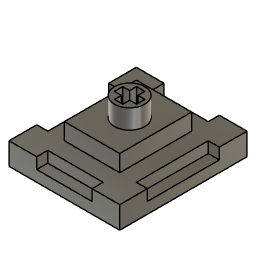
あa (Autodesk Fusion 360 design; units mm, degrees)
Autodesk Fusion 360 part; units mm, degrees
sketch "スケッチ1" plane through (0, 0, 0) normal (0, 0, 1) x (1, 0, 0)
  line L0 (0, 0) -> (20, 0)
  line L1 (20, 0) -> (20, 23)
  line L2 (20, 23) -> (0, 23)
  line L3 (0, 23) -> (0, 0)
  dimension "d1" = 20
  dimension "d2" = 23
  constraint horizontal L0
  constraint vertical L1
  constraint horizontal L2
  constraint vertical L3
  constraint coincident L0.start L3.end
  measures "d1" distance of L0.start L0.end
  measures "d2" distance of L0.start L2.end
extrude "押し出し1" add sketch "スケッチ1" along normal blind 2
sketch "スケッチ2" plane through (0, 0, 2) normal (0, 0, 1) x (-1, 0, 0)
  line L0 (0, -23) -> (0, 0)
  line L1 (0, 0) -> (-20, 0)
  line L2 (-20, 0) -> (-20, -23)
  line L3 (-20, -23) -> (0, -23)
  line L4 (0, -23) -> (-5, -23)
  line L5 (-5, -23) -> (-5, -18)
  line L6 (-5, -18) -> (0, -18)
  line L7 (0, -18) -> (0, -23)
  line L8 (-20, -23) -> (-15, -23)
  line L9 (-15, -23) -> (-15, -18)
  line L10 (-15, -18) -> (-20, -18)
  line L11 (-20, -18) -> (-20, -23)
  line L12 (0, 0) -> (-5, 0)
  line L13 (-5, 0) -> (-5, -5)
  line L14 (-5, -5) -> (0, -5)
  line L15 (0, -5) -> (0, 0)
  line L16 (-20, 0) -> (-15, 0)
  line L17 (-15, 0) -> (-15, -5)
  line L18 (-15, -5) -> (-20, -5)
  line L19 (-20, -5) -> (-20, 0)
  line L20 (-2, -21) -> (-18, -21)
  line L21 (-18, -21) -> (-18, -2)
  line L22 (-18, -2) -> (-2, -2)
  line L23 (-2, -2) -> (-2, -21)
  dimension "d5" = 5
  dimension "d6" = 5
  dimension "d7" = 5
  dimension "d8" = 5
  dimension "d9" = 5
  dimension "d10" = 5
  dimension "d11" = 5
  dimension "d12" = 5
  constraint horizontal L4
  constraint vertical L5
  constraint horizontal L6
  constraint vertical L7
  constraint coincident L0.start L3.end
  constraint horizontal L8
  constraint vertical L9
  constraint horizontal L10
  constraint vertical L11
  constraint coincident L2.end L3.start
  constraint horizontal L12
  constraint vertical L13
  constraint horizontal L14
  constraint vertical L15
  constraint coincident L0.end L1.start
  constraint horizontal L16
  constraint vertical L17
  constraint horizontal L18
  constraint vertical L19
  constraint coincident L1.end L2.start
  constraint horizontal L20
  constraint vertical L21
  constraint horizontal L22
  constraint vertical L23
  measures "d5" distance of L0.start L4.end
  measures "d6" distance of L0.start L6.end
  measures "d7" distance of L2.end L8.end
  measures "d8" distance of L2.end L10.end
  measures "d9" distance of L0.end L12.end
  measures "d10" distance of L0.end L14.end
  measures "d11" distance of L1.end L16.end
  measures "d12" distance of L1.end L18.end
extrude "押し出し2" add sketch "スケッチ2" along normal blind 2 contours L0 L3 L4 L5 L6 L7 L20 L23 | L0 L1 L12 L13 L14 L15 L22 L23 | L5 L6 L20 L23 | L5 L6 L9 L10 L13 L14 L17 L18 L20 L21 L22 L23 | L2 L3 L8 L9 L10 L11 L20 L21 | L13 L14 L22 L23 | L9 L10 L20 L21 | L1 L2 L16 L17 L18 L19 L21 L22 | L17 L18 L21 L22
sketch "スケッチ3" plane through (0, 0, 4) normal (0, 0, 1) x (-1, 0, 0)
  line L0 (-18, -18) -> (-20, -18)
  line L1 (-20, -18) -> (-20, -23)
  line L2 (-20, -23) -> (-15, -23)
  line L3 (-15, -23) -> (-15, -21)
  line L4 (-15, -21) -> (-5, -21)
  line L5 (-5, -21) -> (-5, -23)
  line L6 (-5, -23) -> (0, -23)
  line L7 (0, -23) -> (0, -18)
  line L8 (0, -18) -> (-2, -18)
  line L9 (-2, -18) -> (-2, -5)
  line L10 (-2, -5) -> (0, -5)
  line L11 (0, -5) -> (0, 0)
  line L12 (0, 0) -> (-5, 0)
  line L13 (-5, 0) -> (-5, -2)
  line L14 (-5, -2) -> (-15, -2)
  line L15 (-15, -2) -> (-15, 0)
  line L16 (-15, 0) -> (-20, 0)
  line L17 (-20, 0) -> (-20, -5)
  line L18 (-20, -5) -> (-18, -5)
  line L19 (-18, -5) -> (-18, -18)
  line L20 (-5, -18) -> (-15, -18)
  line L21 (-15, -18) -> (-15, -5)
  line L22 (-15, -5) -> (-5, -5)
  line L23 (-5, -5) -> (-5, -18)
  constraint horizontal L20
  constraint vertical L21
  constraint horizontal L22
  constraint vertical L23
extrude "押し出し3" add sketch "スケッチ3" along normal blind 3 contours L20 L21 L22 L23
sketch "スケッチ4" plane through (0, 0, 7) normal (0, 0, 1) x (-1, 0, 0)
  line L0 (-5, -5) -> (-15, -5)
  line L1 (-15, -5) -> (-15, -18)
  line L2 (-15, -18) -> (-5, -18)
  line L3 (-5, -18) -> (-5, -5)
  line L4 (-9.55, -13.5) -> (-11.05, -13.5)
  line L5 (-11.05, -13.5) -> (-11.05, -9.5)
  line L6 (-11.05, -9.5) -> (-9.55, -9.5)
  line L7 (-9.55, -9.5) -> (-9.55, -13.5)
  line L8 (-8.3, -12.25) -> (-12.3, -12.25)
  line L9 (-12.3, -12.25) -> (-12.3, -10.75)
  line L10 (-12.3, -10.75) -> (-8.3, -10.75)
  line L11 (-8.3, -10.75) -> (-8.3, -12.25)
  circle A0 centre (-10.3, -11.5) radius 2.75
  dimension "d17" = 13
  dimension "d18" = 1.5
  dimension "d19" = 4
  dimension "d20" = 4
  dimension "d21" = 1.5
  dimension "d22" = 5.5
  constraint horizontal L4
  constraint vertical L5
  constraint horizontal L6
  constraint vertical L7
  constraint horizontal L8
  constraint vertical L9
  constraint horizontal L10
  constraint vertical L11
  measures "d17" distance of L0 L2
  measures "d18" distance of L4.start L4.end
  measures "d19" distance of L4.start L6.end
  measures "d20" distance of L8.start L8.end
  measures "d21" distance of L8.start L10.end
  measures "d22" diameter of A0
extrude "押し出し4" add sketch "スケッチ4" along normal blind 3.5 contours A0
sketch "スケッチ5" plane through (0, 0, 0) normal (0, 0, -1) x (1, 0, 0)
  line L0 (0, 0) -> (0, -23)
  line L1 (0, -23) -> (20, -23)
  line L2 (20, -23) -> (20, 0)
  line L3 (20, 0) -> (0, 0)
  line L4 (20, -5) -> (0, -5) construction
  line L5 (0, -5) -> (0, -20) construction
  line L6 (0, -20) -> (20, -20) construction
  line L7 (20, -20) -> (20, -5) construction
  spline S0 degree 2 poles (12.4, -9.2465) (10.8153, -9.4071) (10.308, -9.915) knots 0 0 0 1 1 1
  spline S1 degree 2 poles (10.308, -9.915) (9.9278, -10.2946) (9.9278, -11.0222) knots 0 0 0 1 1 1
  spline S2 degree 2 poles (9.9278, -11.0222) (9.9278, -11.7963) (10.308, -12.1759) knots 0 0 0 1 1 1
  spline S3 degree 2 poles (10.308, -12.1759) (10.7658, -12.6343) (11.4922, -12.7053) knots 0 0 0 1 1 1
  spline S4 degree 2 poles (11.4922, -12.7053) (12.0723, -10.8115) (12.8076, -10.057) knots 0 0 0 1 1 1
  line L8 (12.8076, -10.057) -> (12.5826, -9.5581)
  line L9 (12.5826, -9.5581) -> (13.4558, -8.96)
  line L10 (13.4558, -8.96) -> (13.6391, -9.3718)
  spline S5 degree 2 poles (13.6391, -9.3718) (14.5284, -8.5482) (15.244, -8.5482) knots 0 0 0 1 1 1
  spline S6 degree 2 poles (15.244, -8.5482) (15.7436, -8.5482) (16.1507, -8.9546) knots 0 0 0 1 1 1
  spline S7 degree 2 poles (16.1507, -8.9546) (16.5947, -9.3993) (16.5947, -10.1609) knots 0 0 0 1 1 1
  spline S8 degree 2 poles (16.5947, -10.1609) (16.5947, -11.4555) (15.7012, -12.3496) knots 0 0 0 1 1 1
  spline S9 degree 2 poles (15.7012, -12.3496) (15.179, -12.8712) (14.6454, -13.156) knots 0 0 0 1 1 1
  line L11 (14.6454, -13.156) -> (14.572, -14.4285)
  line L12 (14.572, -14.4285) -> (16.1256, -14.3533)
  line L13 (16.1256, -14.3533) -> (16.2951, -15.3649)
  line L14 (16.2951, -15.3649) -> (14.532, -15.4019)
  spline S10 degree 2 poles (14.532, -15.4019) (14.4974, -16.1982) (14.4156, -17.0535) knots 0 0 0 1 1 1
  line L15 (14.4156, -17.0535) -> (13.5865, -17.0535)
  spline S11 degree 2 poles (13.5865, -17.0535) (13.1073, -16.9341) (13.4141, -16.6136) knots 0 0 0 1 1 1
  spline S12 degree 2 poles (13.4141, -16.6136) (13.4839, -15.9851) (13.5191, -15.4813) knots 0 0 0 1 1 1
  spline S13 degree 2 poles (13.5191, -15.4813) (11.8628, -15.553) (10.4662, -15.8186) knots 0 0 0 1 1 1
  line L16 (10.4662, -15.8186) -> (10.2978, -14.7794)
  spline S14 degree 2 poles (10.2978, -14.7794) (11.9661, -14.5789) (13.5651, -14.5072) knots 0 0 0 1 1 1
  line L17 (13.5651, -14.5072) -> (13.6313, -13.5338)
  spline S15 degree 2 poles (13.6313, -13.5338) (13.2535, -13.6806) (12.3874, -13.7158) knots 0 0 0 1 1 1
  line L18 (12.3874, -13.7158) -> (12.2711, -14.358)
  line L19 (12.2711, -14.358) -> (11.4474, -14.2064)
  spline S16 degree 2 poles (11.4474, -14.2064) (11.0099, -14.0877) (11.2797, -13.7725) knots 0 0 0 1 1 1
  line L20 (11.2797, -13.7725) -> (11.3095, -13.6334)
  spline S17 degree 2 poles (11.3095, -13.6334) (10.1988, -13.5272) (9.5458, -12.8736) knots 0 0 0 1 1 1
  spline S18 degree 2 poles (9.5458, -12.8736) (8.7997, -12.1282) (8.7997, -10.9846) knots 0 0 0 1 1 1
  spline S19 degree 2 poles (8.7997, -10.9846) (8.7997, -9.8875) (9.4706, -9.2173) knots 0 0 0 1 1 1
  spline S20 degree 2 poles (9.4706, -9.2173) (10.1713, -8.5165) (11.858, -8.2486) knots 0 0 0 1 1 1
  line L21 (11.858, -8.2486) -> (12.4, -9.2465)
  spline S21 degree 2 poles (14.523, -12.2183) (14.6525, -12.0876) (15.0136, -11.7265) knots 0 0 0 1 1 1
  spline S22 degree 2 poles (15.0136, -11.7265) (15.6541, -11.086) (15.6541, -10.0487) knots 0 0 0 1 1 1
  spline S23 degree 2 poles (15.6541, -10.0487) (15.6541, -9.7688) (15.4631, -9.5778) knots 0 0 0 1 1 1
  spline S24 degree 2 poles (15.4631, -9.5778) (15.4112, -9.5258) (15.244, -9.5258) knots 0 0 0 1 1 1
  spline S25 degree 2 poles (15.244, -9.5258) (14.7421, -9.5258) (14.0855, -10.1716) knots 0 0 0 1 1 1
  spline S26 degree 2 poles (14.0855, -10.1716) (14.4586, -11.2591) (14.523, -12.2183) knots 0 0 0 1 1 1
  spline S27 degree 2 poles (13.5567, -12.6253) (13.5215, -11.742) (13.263, -10.9494) knots 0 0 0 1 1 1
  spline S28 degree 2 poles (13.263, -10.9494) (12.8094, -11.6769) (12.5498, -12.7805) knots 0 0 0 1 1 1
  spline S29 degree 2 poles (12.5498, -12.7805) (13.0894, -12.7805) (13.5567, -12.6253) knots 0 0 0 1 1 1
  line L22 (6.395, -12.6337) -> (7.6126, -12.8533)
  spline S30 degree 2 poles (7.6126, -12.8533) (7.4072, -13.5887) (6.9059, -13.942) knots 0 0 0 1 1 1
  spline S31 degree 2 poles (6.9059, -13.942) (6.4045, -14.2954) (5.4161, -14.2954) knots 0 0 0 1 1 1
  spline S32 degree 2 poles (5.4161, -14.2954) (4.5184, -14.2954) (4.0791, -14.0829) knots 0 0 0 1 1 1
  spline S33 degree 2 poles (4.0791, -14.0829) (3.6398, -13.8704) (3.4608, -13.5433) knots 0 0 0 1 1 1
  spline S34 degree 2 poles (3.4608, -13.5433) (3.2817, -13.2162) (3.2817, -12.3424) knots 0 0 0 1 1 1
  line L23 (3.2817, -12.3424) -> (3.296, -10.7763)
  spline S35 degree 2 poles (3.296, -10.7763) (3.296, -10.1078) (3.2316, -9.7902) knots 0 0 0 1 1 1
  spline S36 degree 2 poles (3.2316, -9.7902) (3.1671, -9.4727) (2.9905, -9.1098) knots 0 0 0 1 1 1
  line L24 (2.9905, -9.1098) -> (4.3179, -9.1098)
  spline S37 degree 2 poles (4.3179, -9.1098) (4.3704, -9.2435) (4.4468, -9.5061) knots 0 0 0 1 1 1
  spline S38 degree 2 poles (4.4468, -9.5061) (4.4802, -9.6255) (4.4945, -9.6637) knots 0 0 0 1 1 1
  spline S39 degree 2 poles (4.4945, -9.6637) (4.8383, -9.3295) (5.2299, -9.1623) knots 0 0 0 1 1 1
  spline S40 degree 2 poles (5.2299, -9.1623) (5.6214, -8.9952) (6.0655, -8.9952) knots 0 0 0 1 1 1
  spline S41 degree 2 poles (6.0655, -8.9952) (6.8486, -8.9952) (7.2998, -9.4202) knots 0 0 0 1 1 1
  spline S42 degree 2 poles (7.2998, -9.4202) (7.751, -9.8452) (7.751, -10.4945) knots 0 0 0 1 1 1
  spline S43 degree 2 poles (7.751, -10.4945) (7.751, -10.9243) (7.5457, -11.2609) knots 0 0 0 1 1 1
  spline S44 degree 2 poles (7.5457, -11.2609) (7.3404, -11.5975) (6.9703, -11.7766) knots 0 0 0 1 1 1
  spline S45 degree 2 poles (6.9703, -11.7766) (6.6003, -11.9557) (5.9031, -12.0894) knots 0 0 0 1 1 1
  spline S46 degree 2 poles (5.9031, -12.0894) (4.9625, -12.266) (4.5996, -12.4188) knots 0 0 0 1 1 1
  line L25 (4.5996, -12.4188) -> (4.5996, -12.5525)
  spline S47 degree 2 poles (4.5996, -12.5525) (4.5996, -12.9393) (4.7906, -13.104) knots 0 0 0 1 1 1
  spline S48 degree 2 poles (4.7906, -13.104) (4.9816, -13.2688) (5.5116, -13.2688) knots 0 0 0 1 1 1
  spline S49 degree 2 poles (5.5116, -13.2688) (5.8697, -13.2688) (6.0703, -13.1279) knots 0 0 0 1 1 1
  spline S50 degree 2 poles (6.0703, -13.1279) (6.2708, -12.987) (6.395, -12.6337) knots 0 0 0 1 1 1
  spline S51 degree 2 poles (4.5996, -11.545) (4.8574, -11.4591) (5.4161, -11.3397) knots 0 0 0 1 1 1
  spline S52 degree 2 poles (5.4161, -11.3397) (5.9748, -11.2203) (6.1467, -11.1057) knots 0 0 0 1 1 1
  spline S53 degree 2 poles (6.1467, -11.1057) (6.4093, -10.9195) (6.4093, -10.633) knots 0 0 0 1 1 1
  spline S54 degree 2 poles (6.4093, -10.633) (6.4093, -10.3513) (6.1992, -10.146) knots 0 0 0 1 1 1
  spline S55 degree 2 poles (6.1992, -10.146) (5.9891, -9.9407) (5.6644, -9.9407) knots 0 0 0 1 1 1
  spline S56 degree 2 poles (5.6644, -9.9407) (5.3015, -9.9407) (4.972, -10.1794) knots 0 0 0 1 1 1
  spline S57 degree 2 poles (4.972, -10.1794) (4.7285, -10.3608) (4.6521, -10.6235) knots 0 0 0 1 1 1
  spline S58 degree 2 poles (4.6521, -10.6235) (4.5996, -10.7954) (4.5996, -11.2776) knots 0 0 0 1 1 1
  line L26 (4.5996, -11.2776) -> (4.5996, -11.545)
extrude "押し出し5" cut sketch "スケッチ5" against normal blind 1 contours S0 S1 S2 S3 S4 L8 L9 L10 S5 S6 S7 S8 S9 L11 L12 L13 L14 S10 L15 S11 S12 S13 L16 S14 L17 S15 L18 L19 S16 L20 S17 S18 S19 S20 L21 | L22 S30 S31 S32 S33 S34 L23 S35 S36 L24 S37 S38 S39 S40 S41 S42 S43 S44 S45 S46 L25 S47 S48 S49 S50
